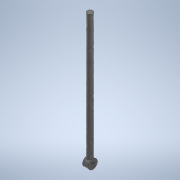
# Autodesk Inventor part: BarX70mm
Saved by Autodesk Inventor 2022 (Build 260153000, 153)
## iProperties
Created: 2021-11-09
Part Number: BarX70mm
Material: Generic
Document SubType Name: Modeling
Designer: Juan
Density: 1 g/cm^3
Appearance: Default
Author: Juan
Autodesk Inventor part; units mm, degrees
ref_plane "YZ Plane" through (0, 0, 0) normal (1, 0, 0) x (0, 1, 0)
sketch "Sketch1" plane through (0, 0, 0) normal (1, 0, 0) x (0, 1, 0)
  circle A0 centre (0, 0) radius 1
  circle A1 centre (0, 0) radius 2.5
  dimension "d0" = 2
  dimension "d1" = 5
  constraints: 2 centre point, 2 coincident
  measures "d0" diameter of A0
  measures "d1" diameter of A1
extrude "Extrusion1" add sketch "Sketch1" along normal blind 3
ref_plane "Work Plane1" through (1.5, 0, 0) normal (1, 0, 0) x (0, 0, -1)
ref_plane "Work Plane2" through (0, 70, 0) normal (0, 1, 0) x (-1, 0, 0)
sketch "Sketch2" plane through (0, 70, 0) normal (0, 1, 0) x (-1, 0, 0)
  line L0 (0, 2.5) -> (0, -2.5) projected
  point P0 (0, 0)
sketch "Sketch3" plane through (0, 70, 0) normal (0, 1, 0) x (-1, 0, 0)
  line L0 (0, 0) -> (-1.5, 0)
  circle A0 centre (-1.5, 0) radius 1.5
  dimension "d5" = 1.5
  dimension "d6" = 3
  constraints: 2 end point, 1 centre point, 1 coincident, 1 horizontal
  measures "d5" distance of L0.start L0.end
  measures "d6" diameter of A0
extrude "Extrusion2" add sketch "Sketch3" against normal up to surface
body "Solid1"
